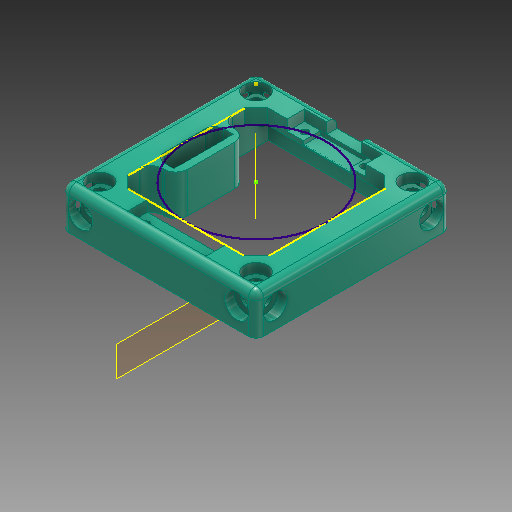
# Autodesk Inventor part: 10_Lid_el_v0
Saved by Autodesk Inventor 2019 (Build 230136000, 136)
## iProperties
Created: 2018-05-19
Part Number: 10_Lid_el_v0
Material: Generisch
Document SubType Name: Modeling
Designer: diederichbenedict
Density: 1 g/cm^3
Appearance: IPHT_Türkis
Mass: 9.15968 g
Surface Area: 74.6558 cm^2
Volume: 9.15968 cm^3
Author: diederichbenedict
Autodesk Inventor part; units mm, degrees
ref_plane "YZ Plane" through (0, 0, 0) normal (1, 0, 0) x (0, 1, 0)
sketch "Skizze1" plane through (0, 0, 0) normal (0, 0, 1) x (1, 0, 0)
  line L0 (-3.2746, 3.2746) -> (46.5254, 3.2746)
  line L1 (46.5254, 3.2746) -> (46.5254, -46.5254)
  line L2 (46.5254, -46.5254) -> (-3.2746, -46.5254)
  line L3 (-3.2746, -46.5254) -> (-3.2746, 3.2746)
  line L4 (-3.2746, 3.2746) -> (46.5254, -46.5254) construction
  line L5 (46.5254, 3.2746) -> (-3.2746, -46.5254) construction
  line L6 (6.7254, -3.7254) -> (36.5254, -3.7254)
  line L7 (39.5254, -6.7254) -> (39.5254, -36.5254)
  line L8 (36.5254, -39.5254) -> (6.7254, -39.5254)
  line L9 (3.7254, -36.5254) -> (3.7254, -6.7254)
  line L10 (3.7254, -3.7254) -> (39.5254, -39.5254) construction
  line L11 (39.5254, -3.7254) -> (3.7254, -39.5254) construction
  line L12 (36.5254, -39.5254) -> (39.5254, -36.5254)
  line L13 (6.7254, -39.5254) -> (3.7254, -36.5254)
  line L14 (3.7254, -6.7254) -> (6.7254, -3.7254)
  line L15 (36.5254, -3.7254) -> (39.5254, -6.7254)
  line L16 (6.9985, -0.5594) -> (36.2523, -0.5594) projected
  line L17 (36.2523, -0.5594) -> (36.2523, 3.2746) projected
  line L18 (36.2523, 3.2746) -> (6.9985, 3.2746) projected
  line L19 (6.9985, 3.2746) -> (6.9985, -0.5594) projected
  point P0 (21.6254, -21.6254)
  point P1 (21.6254, -21.6254)
  dimension "d17" = 35.8
  dimension "d18" = 35.8
  dimension "d19" = 3
  dimension "d20" = 3
  dimension "d21" = 3
  dimension "d22" = 3
  dimension "d23" = 3
  dimension "d24" = 3
  dimension "d25" = 3
  dimension "d26" = 3
  constraints: 32 end point, 8 point on line, 5 midpoint, 4 parallel, 2 horizontal, 2 perpendicular
  measures "d17" distance of L10.end L11.end
  measures "d18" distance of L11.start L10.end
  measures "d19" distance of L8.start L10.end
  measures "d20" distance of L7.end L10.end
  measures "d21" distance of L8.end L11.end
  measures "d22" distance of L9.start L11.end
  measures "d23" distance of L9.end L10.start
  measures "d24" distance of L6.start L10.start
  measures "d25" distance of L6.end L11.start
  measures "d26" distance of L7.start L11.start
extrude "Extrusion1" add sketch "Skizze1" along normal blind 10.3
sketch "Skizze2" plane through (0, 0, 10.3) normal (0, 0, 1) x (1, 0, 0)
  arc A0 (41.4389, -3.1137) -> (40.137, -1.8118) centre (41.6254, -1.6254) ccw projected
  arc A1 (40.137, -41.4389) -> (41.4389, -40.137) centre (41.6254, -41.6254) ccw projected
  arc A2 (1.8118, -40.137) -> (3.1137, -41.4389) centre (1.6254, -41.6254) ccw projected
  arc A3 (3.1137, -1.8118) -> (1.8118, -3.1137) centre (1.6254, -1.6254) ccw projected
hole "Bohrung1" at (41.6254, -41.6254, 10.3) at (1.6254, -41.6254, 10.3) at (1.6254, -1.6254, 10.3) at (41.6254, -1.6254, 10.3) direction (0, 0, -1) diameter 3.2 end through all counterbore diameter 6 counterbore depth 2.5
fillet "Rundung1" radius 2 8 edges at (21.6254, -46.5254, 10.3) (-3.2746, -21.6254, 10.3) (21.6254, 3.2746, 10.3) (46.5254, -21.6254, 10.3) (46.5254, 3.2746, 5.15) (46.5254, -46.5254, 5.15) (-3.2746, -46.5254, 5.15) (-3.2746, 3.2746, 5.15)
sketch "Skizze3" plane through (-1.2746, -46.5254, 0) normal (0, -1, 0) x (1, 0, 0)
  line L0 (2.119, -37.7) -> (0, -37.7) construction
  line L1 (42.9, -36) -> (2.9, -36) construction
  line L2 (2.9, -36) -> (2.9, 5.3) construction
  line L3 (2.9, 5.3) -> (42.9, 5.3) construction
  line L4 (42.9, 5.3) -> (42.9, -36) construction
  arc A0 (0, -35.7954) -> (2.119, -37.7) centre (2.9, -34.7) ccw projected
  line L5 (0, -37.7) -> (0, -35.7954) projected
  dimension "d40" = 40
  constraints: 8 end point, 2 parallel, 1 horizontal, 1 perpendicular
  measures "d40" distance of L2.end L3.end
sketch "Skizze4" plane through (0, 0, 10.3) normal (0, 0, 1) x (1, 0, 0)
  line L0 (36.5254, -39.5254) -> (6.7254, -39.5254) projected
  line L1 (39.5254, -6.7254) -> (39.5254, -36.5254) projected
  line L2 (3.7254, -36.5254) -> (3.7254, -6.7254) projected
  circle A0 centre (21.6254, -21.6254) radius 17.9
  point P0 (0, 0)
  constraints: 3 tangent, 1 centre point
ref_plane "Arbeitsebene1" through (3.7254, -5.5842, -33.1) normal (1, 0, 0) x (0, 1, 0)
sketch "Skizze5" plane through (3.7254, -5.5842, -33.1) normal (1, 0, 0) x (0, 1, 0)
  line L0 (-36.1071, 36.3288) -> (-36.1071, 0.4712) construction
  line L1 (-36.1071, 0.4712) -> (-33.9699, -1.666) construction
  line L2 (-33.9699, -1.666) -> (1.8877, -1.666) construction
  line L3 (1.8877, -1.666) -> (4.0249, 0.4712) construction
  line L4 (4.0249, 0.4712) -> (4.0249, 36.3288) construction
  line L5 (4.0249, 36.3288) -> (1.8877, 38.466) construction
  line L6 (1.8877, 38.466) -> (-33.9699, 38.466) construction
  line L7 (-33.9699, 38.466) -> (-36.1071, 36.3288) construction
  circle A0 centre (-1.0412, 3.4) radius 3.2639 construction
  circle A1 centre (-31.0411, 3.4) radius 3.2639 construction
  circle A2 centre (-1.0412, 33.4) radius 3.2639 construction
  circle A3 centre (-31.0411, 33.4) radius 3.2639 construction
  circle A4 centre (-16.0411, 18.4) radius 13.3985 construction
  line L8 (-34.3841, -2.666) -> (-37.1071, 0.057)
  line L9 (-37.1071, 0.057) -> (-37.1071, 36.743)
  line L10 (-37.1071, 36.743) -> (-34.3841, 39.466)
  line L11 (-34.3841, 39.466) -> (2.3019, 39.466)
  line L12 (2.3019, 39.466) -> (5.0249, 36.743)
  line L13 (5.0249, 36.743) -> (5.0249, 0.057)
  line L14 (5.0249, 0.057) -> (2.3019, -2.666)
  line L15 (2.3019, -2.666) -> (-34.3841, -2.666)
  point P0 (5.5842, 33.1)
  dimension "d27" = 1
  constraints: 16 end point, 7 other
  measures "d27" distance between parallel lines of L1 L8
ref_plane "Arbeitsebene2" through (39.5254, -37.6665, -43) normal (-1, 0, 0) x (0, 0, 1)
extrude "Extrusion3" cut sketch "Skizze5" along normal up to surface (35.8 mm away)
hole "Bohrung2" at (41.6254, -46.5254, 5.3) at (1.6254, -46.5254, 5.3) direction (0, 1, 0) diameter 3.2 depth 15 tip angle 118 counterbore diameter 6.2 counterbore depth 2.5
pattern_circular "Runde Anordnung2" count 4 over 360 about axis through (21.6254, -21.6254, 10.3) along (0, 0, 1) of "Bohrung2"
sketch "Skizze6" plane through (0, 0, 0) normal (0, 0, -1) x (-1, 0, 0)
  line L0 (-8.1873, -15.1254) -> (-7.1873, -15.1254) construction
  line L1 (-7.1873, -15.1254) -> (-7.1873, -28.1254) construction
  line L2 (-7.1873, -28.1254) -> (-8.1873, -28.1254) construction
  line L3 (-8.1873, -28.1254) -> (-8.1873, -29.1254) construction
  line L4 (-8.1873, -29.1254) -> (-5.8373, -29.1254) construction
  arc A0 (-5.8373, -29.1254) -> (-3.4873, -26.7754) centre (-5.8373, -26.7754) ccw construction
  line L5 (-3.4873, -26.7754) -> (-3.4873, -16.4754) construction
  arc A1 (-3.4873, -16.4754) -> (-5.8373, -14.1254) centre (-5.8373, -16.4754) ccw construction
  line L6 (-5.8373, -14.1254) -> (-8.1873, -14.1254) construction
  line L7 (-8.1873, -14.1254) -> (-8.1873, -15.1254) construction
  line L8 (-3.7254, -36.5254) -> (-3.7254, -6.7254) projected
  line L9 (-10.1254, -12.6254) -> (-3.7254, -12.6254)
  line L10 (-3.7254, -12.6254) -> (-3.7254, -30.6254)
  line L11 (-3.7254, -30.6254) -> (-10.1254, -30.6254)
  line L12 (-10.1254, -30.6254) -> (-10.1254, -12.6254)
  line L13 (-13.0254, -4.1254) -> (-6.1254, -4.1254) projected
  line L14 (3.3746, 3.3746) -> (-13.0254, 3.3746) projected
  line L15 (3.3746, -13.0254) -> (3.3746, 3.3746) projected
  line L16 (-13.0254, -4.1254) -> (-13.0254, 3.3746) projected
  arc A2 (-4.1254, -6.1254) -> (-6.1254, -4.1254) centre (-6.1254, -6.1254) ccw projected
  line L17 (-4.1254, -6.1254) -> (-4.1254, -13.0254) projected
  line L18 (3.3746, -13.0254) -> (-4.1254, -13.0254) projected
  circle A3 centre (-1.6254, -1.6254) radius 2.2989 projected
  point P0 (0, 0)
  constraints: 8 end point, 2 parallel, 1 horizontal, 1 perpendicular, 1 point on line
extrude "Extrusion4" add sketch "Skizze6" against normal up to surface (10.3 mm away) contours L11 L12 L9 L17 L18 L8 | L18 L17 L9 L8
fillet "Rundung2" radius 3 4 edges at (3.7254, -30.6254, 5.15) (10.1254, -30.6254, 5.15) (10.1254, -12.6254, 5.15) (3.7254, -12.6254, 5.15)
sketch "Skizze7" plane through (0, 0, 0) normal (0, 0, -1) x (-1, 0, 0)
  arc A0 (-8.6873, -26.3754) -> (-5.8373, -29.2254) centre (-5.8373, -26.3754) ccw construction
  arc A1 (-5.8373, -14.0254) -> (-8.6873, -16.8754) centre (-5.8373, -16.8754) ccw construction
  arc A2 (-3.4873, -16.4754) -> (-5.8373, -14.1254) centre (-5.8373, -16.4754) ccw construction
  arc A3 (-5.8373, -29.1254) -> (-3.4873, -26.7754) centre (-5.8373, -26.7754) ccw construction
  line L0 (-8.1873, -15.1254) -> (-8.1873, -28.1254) construction
  line L1 (-5.8373, -14.0254) -> (-5.8373, -29.2254) construction
  line L2 (-3.4373, -16.4254) -> (-3.4373, -26.8254)
  line L3 (-8.2373, -26.8254) -> (-8.2373, -16.4254)
  arc A4 (-3.4373, -16.4254) -> (-8.2373, -16.4254) centre (-5.8373, -16.4254) ccw
  arc A5 (-8.2373, -26.8254) -> (-3.4373, -26.8254) centre (-5.8373, -26.8254) ccw
  line L4 (-5.8373, -14.0254) -> (-8.1873, -14.0254)
  line L5 (-8.1873, -14.0254) -> (-8.1873, -29.2254)
  line L6 (-8.1873, -29.2254) -> (-5.8373, -29.2254)
  line L7 (-5.8373, -29.2254) -> (-5.8373, -14.0254)
  point P0 (0, 0)
  point P1 (-5.8373, -21.6254)
  point P2 (-8.1873, -21.6254)
  dimension "d48" = 4.8
  constraints: 16 end point, 6 point on circle, 4 tangent, 3 midpoint, 3 parallel, 2 centre point, 2 point on line, 1 horizontal, 1 perpendicular, 1 vertical
  measures "d48" distance between parallel lines of L3 L2
extrude "Extrusion5" cut sketch "Skizze7" against normal through all
sketch "Skizze8" plane through (0, 0, 10.3) normal (0, 0, 1) x (1, 0, 0)
  line L0 (12.7254, -43.5254) -> (30.7254, -43.5254) construction
  line L1 (30.7254, -43.5254) -> (30.7254, -0.3254) construction
  line L2 (30.7254, -0.3254) -> (12.7254, -0.3254) construction
  line L3 (12.7254, -0.3254) -> (12.7254, -43.5254) construction
  circle A0 centre (19.1854, -42.1184) radius 0.5 construction
  circle A1 centre (24.2654, -42.1184) radius 0.5 construction
  circle A2 centre (21.7254, -39.5784) radius 0.5 construction
  circle A3 centre (29.3454, -1.6054) radius 0.9 construction
  circle A4 centre (14.1054, -42.2454) radius 0.9 construction
  circle A5 centre (19.5254, -4.3754) radius 0.4 construction
  circle A6 centre (23.9254, -4.3754) radius 0.4 construction
  circle A7 centre (14.1054, -4.1454) radius 0.9 construction
  circle A8 centre (14.1054, -6.6854) radius 0.9 construction
  circle A9 centre (14.1054, -9.2254) radius 0.9 construction
  circle A10 centre (14.1054, -11.7654) radius 0.9 construction
  circle A11 centre (14.1054, -14.3054) radius 0.9 construction
  circle A12 centre (14.1054, -16.8454) radius 0.9 construction
  circle A13 centre (14.1054, -19.3854) radius 0.9 construction
  circle A14 centre (14.1054, -21.9254) radius 0.9 construction
  circle A15 centre (14.1054, -24.4654) radius 0.9 construction
  circle A16 centre (14.1054, -27.0054) radius 0.9 construction
  circle A17 centre (14.1054, -29.5454) radius 0.9 construction
  circle A18 centre (14.1054, -32.0854) radius 0.9 construction
  circle A19 centre (14.1054, -34.6254) radius 0.9 construction
  circle A20 centre (14.1054, -37.1654) radius 0.9 construction
  circle A21 centre (14.1054, -39.7054) radius 0.9 construction
  circle A22 centre (29.3454, -4.1454) radius 0.9 construction
  circle A23 centre (29.3454, -6.6854) radius 0.9 construction
  circle A24 centre (29.3454, -9.2254) radius 0.9 construction
  circle A25 centre (29.3454, -11.7654) radius 0.9 construction
  circle A26 centre (29.3454, -14.3054) radius 0.9 construction
  circle A27 centre (29.3454, -16.8454) radius 0.9 construction
  circle A28 centre (29.3454, -19.3854) radius 0.9 construction
  circle A29 centre (29.3454, -21.9254) radius 0.9 construction
  circle A30 centre (29.3454, -24.4654) radius 0.9 construction
  circle A31 centre (29.3454, -27.0054) radius 0.9 construction
  circle A32 centre (29.3454, -29.5454) radius 0.9 construction
  circle A33 centre (29.3454, -32.0854) radius 0.9 construction
  circle A34 centre (29.3454, -34.6254) radius 0.9 construction
  circle A35 centre (29.3454, -37.1654) radius 0.9 construction
  circle A36 centre (29.3454, -39.7054) radius 0.9 construction
  circle A37 centre (29.3454, -42.2454) radius 0.9 construction
  circle A38 centre (14.1054, -1.6054) radius 0.9 construction
  circle A39 centre (24.2654, -39.5784) radius 0.5 construction
  circle A40 centre (21.7254, -42.1184) radius 0.5 construction
  circle A41 centre (19.1854, -39.5784) radius 0.5 construction
  line L4 (11.7254, -44.5254) -> (31.7254, -44.5254)
  line L5 (31.7254, -44.5254) -> (31.7254, 0.6746)
  line L6 (31.7254, 0.6746) -> (11.7254, 0.6746)
  line L7 (11.7254, 0.6746) -> (11.7254, -44.5254)
  line L8 (17.4066, 0.6746) -> (26.2901, 0.6746)
  line L9 (26.2901, 0.6746) -> (26.2901, 4.6302)
  line L10 (26.2901, 4.6302) -> (17.4066, 4.6302)
  line L11 (17.4066, 4.6302) -> (17.4066, 0.6746)
  point P0 (0, 0)
  dimension "d49" = 1
  constraints: 16 end point, 2 parallel, 1 horizontal, 1 perpendicular, 1 point on line, 3 other
  measures "d49" distance between parallel lines of L3 L7
ref_plane "Arbeitsebene3" through (12.7254, -43.5254, 7.55) normal (0, 0, -1) x (0, 1, 0)
extrude "Extrusion6" cut sketch "Skizze8" against normal up to surface (2.75 mm away)
sketch "Skizze9" plane through (11.7254, -39.5254, 7.55) normal (0, 0, 1) x (1, 0, 0)
  circle A0 centre (2.38, -2.72) radius 0.9 projected
  circle A1 centre (17.62, -2.72) radius 0.9 projected
  circle A2 centre (2.38, 37.92) radius 0.9 projected
  circle A3 centre (17.62, 37.92) radius 0.9 projected
  point P0 (-11.7254, 39.5254)
extrude "Extrusion7" cut sketch "Skizze9" against normal blind 10
sketch "Skizze10" plane through (11.7254, -39.5254, 7.55) normal (0, 0, 1) x (1, 0, 0)
  circle A0 centre (2.38, -2.72) radius 0.9 projected
  circle A1 centre (17.62, -2.72) radius 0.9 projected
  line L0 (0, 0) -> (20, 0) projected
  line L1 (0, 0) -> (0, -5) projected
  line L2 (0, -5) -> (20, -5) projected
  line L3 (20, -5) -> (20, 0) projected
  circle A2 centre (2.38, 37.92) radius 0.9 projected
  circle A3 centre (17.62, 37.92) radius 0.9 projected
  line L4 (20, 35.8) -> (0, 35.8) projected
  line L5 (20, 35.8) -> (20, 40.2) projected
  line L6 (20, 40.2) -> (14.5648, 40.2) projected
  line L7 (14.5648, 40.2) -> (14.5648, 42.8) projected
  line L8 (5.6812, 42.8) -> (14.5648, 42.8) projected
  line L9 (5.6812, 42.8) -> (5.6812, 40.2) projected
  line L10 (5.6812, 40.2) -> (0, 40.2) projected
  line L11 (0, 40.2) -> (0, 35.8) projected
  line L12 (16.123, 40.17) -> (4.123, 40.17)
  line L13 (4.123, 40.17) -> (4.123, 35.67)
  line L14 (4.123, 35.67) -> (16.123, 35.67)
  line L15 (16.123, 35.67) -> (16.123, 40.17)
  line L16 (16.123, 40.17) -> (4.123, 35.67) construction
  line L17 (4.123, 40.17) -> (16.123, 35.67) construction
  point P0 (-11.7254, 39.5254)
  point P1 (10.123, 37.92)
  dimension "d54" = 12
  dimension "d55" = 4.5
  constraints: 12 end point, 2 midpoint, 2 parallel, 1 horizontal, 1 perpendicular
  measures "d54" distance of L14.end L13.end
  measures "d55" distance between parallel lines of L12 L14
extrude "Extrusion8" cut sketch "Skizze10" against normal blind 1 contours L15 L14 L13 L4 | L4 L13 L12 L15
equation "\"d20\" = d19"
equation "\"d21\" = d19"
equation "\"d22\" = d21"
equation "\"d23\" = d19"
equation "\"d24\" = d23"
equation "\"d25\" = d19"
equation "\"d26\" = d25"
